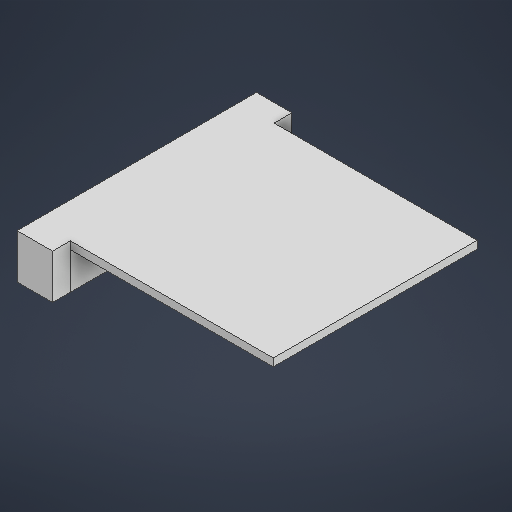
# Autodesk Inventor part: compartment 1
Saved by Autodesk Inventor 2027 (Build 310192060, 192F)
## iProperties
Created: 2026-06-06
Part Number: compartment 1
Material: Generic
Document SubType Name: Modeling
Designer: CatKartikSUPREMEPC
Density: 1 g/cm^3
Appearance: Default
Author: CatKartikSUPREMEPC
Autodesk Inventor part; units mm, degrees
ref_plane "YZ Plane" through (0, 0, 0) normal (1, 0, 0) x (0, 1, 0)
ref_plane "XZ Plane" through (0, 0, 0) normal (0, 1, 0) x (-1, 0, 0)
ref_plane "XY Plane" through (0, 0, 0) normal (0, 0, 1) x (1, 0, 0)
sketch "Sketch1" plane through (0, 0, 0) normal (0, 1, 0) x (-1, 0, 0)
  line L0 (10, -57.295) -> (-10, -57.295)
  line L1 (-10, -57.295) -> (-10, 57.295)
  line L2 (-10, 57.295) -> (10, 57.295)
  line L3 (10, 57.295) -> (10, -57.295)
  line L4 (10, -57.295) -> (-10, 57.295) construction
  line L5 (-10, -57.295) -> (10, 57.295) construction
  point P0 (0, 0)
  dimension "d0" = 114.59
  dimension "d1" = 20
  constraints: 12 end point, 2 midpoint, 2 parallel, 1 horizontal, 1 perpendicular
  measures "d0" distance of L0.end L1.end
  measures "d1" distance between parallel lines of L1 L3
extrude "Extrusion1" add sketch "Sketch1" along normal blind 25
sketch "Sketch2" plane through (10, 0, 57.295) normal (1, 0, 0) x (0, 0, -1)
  line L0 (0, 0) -> (0, 25) projected
  line L1 (114.59, 0) -> (114.59, 25) projected
  line L2 (0, 25) -> (114.59, 25)
  line L3 (114.59, 25) -> (114.59, 20.6952)
  line L4 (114.59, 20.6952) -> (0, 20.6952)
  line L5 (0, 20.6952) -> (0, 25)
  point P0 (57.295, 0)
  constraints: 8 end point, 2 parallel, 1 horizontal, 1 perpendicular, 1 point on line
extrude "Extrusion2" add sketch "Sketch2" along normal blind 114
sketch "Sketch3" plane through (0, 0, 0) normal (0, -1, 0) x (1, 0, 0)
  circle A0 centre (0, 0) radius 6
  circle A1 centre (0, -56.1484) radius 6
  circle A2 centre (0, 56.972) radius 6
  dimension "d7" = 12
  dimension "d9" = 12
  dimension "d10" = 12
  constraints: 3 centre point, 1 coincident
  measures "d7" diameter of A0
  measures "d9" diameter of A1
  measures "d10" diameter of A2
sketch "Sketch4" plane through (-10, 0, 57.295) normal (0, 0, 1) x (1, 0, 0)
  line L0 (20, 0) -> (0, 0) projected
  line L1 (0, 25) -> (134, 25) projected
  line L2 (0, 0) -> (19.9687, 0)
  line L3 (19.9687, 0) -> (19.9687, 25)
  line L4 (19.9687, 25) -> (0, 25)
  line L5 (0, 25) -> (0, 0)
  point P0 (10, 0)
  point P1 (0, 25)
  constraints: 8 end point, 2 parallel, 1 horizontal, 1 perpendicular, 1 point on line
extrude "Extrusion3" add sketch "Sketch4" along normal blind 10
sketch "Sketch5" plane through (10, 0, -57.295) normal (0, 0, -1) x (-1, 0, 0)
  line L0 (20, 0) -> (20, 25) projected
  line L1 (20, 25) -> (-114, 25) projected
  line L2 (20, 0) -> (0.0765, 0)
  line L3 (0.0765, 0) -> (0.0765, 25)
  line L4 (0.0765, 25) -> (20, 25)
  line L5 (20, 25) -> (20, 0)
  point P0 (10, 0)
  constraints: 8 end point, 2 parallel, 1 horizontal, 1 perpendicular, 1 point on line
extrude "Extrusion4" add sketch "Sketch5" along normal blind 10
extrude "Extrusion5" cut sketch "Sketch3" against normal blind 3
body "Solid1"
